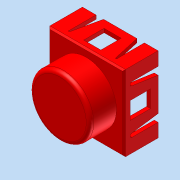
# Autodesk Inventor part: button_cap
Saved by Autodesk Inventor 2014 (Build 180170000, 170)
## iProperties
Created: 2013-01-29
Part Number: button_cap
Document SubType Name: Modeling
Designer: Administrator
Density: 1 g/cm^3
Mass: 0.277875 g
Surface Area: 5.60422 cm^2
Volume: 0.277875 cm^3
Material: Generic
Appearance: Red
Author: Administrator
Autodesk Inventor part; units mm, degrees
ref_plane "YZ Plane" through (0, 0, 0) normal (1, 0, 0) x (0, 1, 0)
ref_plane "XZ Plane" through (0, 0, 0) normal (0, 1, 0) x (-1, 0, 0)
ref_plane "XY Plane" through (0, 0, 0) normal (0, 0, 1) x (1, 0, 0)
sketch "Sketch1" plane through (0, 0, 0) normal (0, 0, 1) x (1, 0, 0)
  line L0 (0, 0) -> (10, 0)
  line L1 (10, 0) -> (10, 10)
  line L2 (10, 10) -> (0, 10)
  line L3 (0, 10) -> (0, 0)
  dimension "d0" = 10
  dimension "d1" = 10
  constraints: 8 end point, 2 parallel, 1 perpendicular, 1 vertical
  measures "d0" distance of L1.end L2.end
  measures "d1" distance of L0.end L1.end
extrude "Extrusion1" add sketch "Sketch1" along normal blind 4.5
sketch "Sketch2" plane through (0, 0, 0) normal (0, -1, 0) x (1, 0, 0)
  line L0 (0, 0) -> (0, 4.5) projected
  line L1 (0, 0) -> (10, 0) projected
  line L2 (10, 0) -> (10, 4.5) projected
  line L3 (1.8, 0) -> (1.8, 3.6067)
  line L4 (2.8, 0) -> (1.9843, 3.6272)
  line L5 (7.2, 0) -> (8.0157, 3.6272)
  line L6 (8.2, 3.6067) -> (8.2, 0)
  arc A0 (1.9843, 3.6272) -> (1.8, 3.6067) centre (1.8933, 3.6067) ccw
  arc A1 (8.2, 3.6067) -> (8.0157, 3.6272) centre (8.1067, 3.6067) ccw
  line L7 (0, 3.7) -> (10, 3.7) construction
  line L8 (3.862, 3.7) -> (6.138, 3.7)
  line L9 (6.138, 3.7) -> (6.138, 1)
  line L10 (6.138, 1) -> (3.862, 1)
  line L11 (3.862, 1) -> (3.862, 3.7)
  dimension "d9" = 1
  dimension "d10" = 1
  dimension "d11" = 3.7
  dimension "d12" = 4.4
  dimension "d13" = 1.8
  dimension "d14" = 1.8
  dimension "d15" = 3.862
  dimension "d16" = 3.862
  dimension "d17" = 1
  constraints: 18 end point, 6 point on line, 6 tangent, 4 point on circle, 4 vertical, 3 horizontal, 2 centre point, 1 collinear, 1 equal radius
  measures "d9" distance of L4.start L3.start
  measures "d10" distance of L6.end L5.start
  measures "d11" distance between parallel lines of L1 L7
  measures "d12" distance of L5.start L4.start
  measures "d13" distance between parallel lines of L0 L3
  measures "d14" distance between parallel lines of L2 L6
  measures "d15" distance between parallel lines of L0 L11
  measures "d16" distance between parallel lines of L2 L9
  measures "d17" distance between parallel lines of L1 L10
extrude "Extrusion2" cut sketch "Sketch2" against normal through all
sketch "Sketch3" plane through (0, 0, 0) normal (-1, 0, 0) x (0, 0, 1)
  line L0 (0, 10) -> (4.5, 10) projected
  line L1 (0, 10) -> (0, 0) projected
  line L2 (0, 0) -> (4.5, 0) projected
  line L3 (0, 10) -> (4.2679, 10)
  line L4 (0, 10) -> (0, 0)
  line L5 (0, 0) -> (4.0987, 0)
  line L6 (0, 8.2) -> (3.4545, 8.2)
  line L7 (0, 7.2) -> (3.4901, 7.7116)
  line L8 (0, 2.8) -> (3.4901, 2.2884)
  line L9 (3.4545, 1.8) -> (0, 1.8)
  arc A0 (3.4901, 7.7116) -> (3.4545, 8.2) centre (3.4545, 7.9545) ccw
  arc A1 (3.4545, 1.8) -> (3.4901, 2.2884) centre (3.4545, 2.0455) ccw
  line L10 (3.7, 10) -> (3.7, 0) construction
  line L11 (3.7, 6.138) -> (3.7, 3.862)
  line L12 (3.7, 3.862) -> (1, 3.862)
  line L13 (1, 3.862) -> (1, 6.138)
  line L14 (1, 6.138) -> (3.7, 6.138)
  dimension "d20" = 1
  dimension "d21" = 1
  dimension "d22" = 3.7
  dimension "d23" = 4.4
  dimension "d24" = 1.8
  dimension "d25" = 1.8
  dimension "d26" = 3.862
  dimension "d27" = 3.862
  dimension "d28" = 1
  constraints: 24 end point, 6 point on line, 6 tangent, 4 collinear, 4 point on circle, 2 centre point, 1 equal radius
  measures "d20" distance of L7.start L6.start
  measures "d21" distance of L9.end L8.start
  measures "d22" distance between parallel lines of L4 L10
  measures "d23" distance of L8.start L7.start
  measures "d24" distance between parallel lines of L3 L6
  measures "d25" distance between parallel lines of L5 L9
  measures "d26" distance between parallel lines of L3 L14
  measures "d27" distance between parallel lines of L5 L12
  measures "d28" distance between parallel lines of L4 L13
extrude "Extrusion3" cut sketch "Sketch3" against normal through all
sketch "Sketch4" plane through (0, 0, 0) normal (0, 0, -1) x (-1, 0, 0)
  line L0 (-2.8, 7.2) -> (-7.2, 7.2) projected
  line L1 (-7.2, 7.2) -> (-7.2, 2.8) projected
  line L2 (-7.2, 2.8) -> (-2.8, 2.8) projected
  line L3 (-2.8, 2.8) -> (-2.8, 7.2) projected
  line L4 (-0.5, 9.5) -> (-9.5, 9.5)
  line L5 (-9.5, 9.5) -> (-9.5, 0.5)
  line L6 (-9.5, 0.5) -> (-0.5, 0.5)
  line L7 (-0.5, 0.5) -> (-0.5, 9.5)
  line L8 (-2.8, 7.2) -> (-7.2, 2.8) construction
  line L9 (-5, 7.2) -> (-5, 2.8) construction
  line L10 (-2.8, 5) -> (-7.2, 5) construction
  point P0 (0, 0)
  dimension "d32" = 4.5
  dimension "d33" = 4.5
  dimension "d34" = 4.5
  constraints: 14 end point, 4 midpoint, 3 equal length, 1 perpendicular
  measures "d32" distance between parallel lines of L7 L9
  measures "d33" distance between parallel lines of L4 L10
  measures "d34" distance between parallel lines of L9 L5
extrude "Extrusion4" cut sketch "Sketch4" against normal blind 4 contours L3 L2 L1 L0 | L7 L6 L5 L4
sketch "Sketch5" plane through (0, 0, 4.5) normal (0, 0, 1) x (1, 0, 0)
  line L0 (0, 0) -> (0, 10) projected
  line L1 (0, 10) -> (10, 10) projected
  circle A0 centre (5, 5) radius 4
  dimension "d37" = 5
  dimension "d38" = 5
  dimension "d39" = 8
  constraints: 1 centre point
  measures "d37" distance from line of L0 A0.centre
  measures "d38" distance from line of L1 A0.centre
  measures "d39" diameter of A0
extrude "Extrusion5" add sketch "Sketch5" along normal blind 3.5
fillet "Fillet1" radius 0.5 1 edges at (1, 5, 8)
chamfer "Chamfer1" distance 0.2 angle 45 4 edges at (5, 10, 4.5) (0, 5, 4.5) (10, 5, 4.5) (5, 0, 4.5)
equation "\"d13\" = d14"
equation "\"d15\" = d16"
equation "\"d24\" = d25"
equation "\"d26\" = d27"
equation "\"d33\" = d32"
equation "\"d34\" = d32"
body "Solid1"
